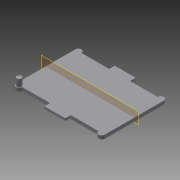
# Autodesk Inventor part: BaseTI stage insert
Saved by Autodesk Inventor 2013 (Build 170138000, 138)
## iProperties
Created: 2012-08-01
Part Number: BaseTI stage insert
Material: Generic
Document SubType Name: Modeling
Designer: kthorn
Density: 1 g/cm^3
Author: kthorn
Autodesk Inventor part; units mm, degrees
ref_plane "YZ Plane" through (0, 0, 0) normal (1, 0, 0) x (0, 1, 0)
ref_plane "XZ Plane" through (0, 0, 0) normal (0, 1, 0) x (-1, 0, 0)
ref_plane "XY Plane" through (0, 0, 0) normal (0, 0, 1) x (1, 0, 0)
sketch "Sketch1" plane through (0, 0, 0) normal (0, 0, 1) x (1, 0, 0)
  line L0 (-54.75, 42.4) -> (54.75, 42.4)
  line L1 (63.55, 42.4) -> (63.55, -42.4)
  line L2 (54.75, -42.4) -> (-54.75, -42.4)
  line L3 (-63.55, -42.4) -> (-63.55, 42.4)
  line L4 (-63.55, 42.4) -> (63.55, -42.4) construction
  line L5 (63.55, 42.4) -> (-63.55, -42.4) construction
  arc A0 (63.55, 42.4) -> (54.75, 42.4) centre (59.15, 42.4) ccw
  line L6 (-63.55, 0) -> (63.55, 0) construction
  line L7 (-8.8, 42.4) -> (-8.8, -42.4) construction
  line L8 (-63.55, 42.4) -> (-54.75, 42.4) construction
  line L9 (-54.75, 42.4) -> (-54.75, 42.4) construction
  arc A1 (-63.55, -42.4) -> (-54.75, -42.4) centre (-59.15, -42.4) ccw
  arc A2 (54.75, -42.4) -> (63.55, -42.4) centre (59.15, -42.4) ccw
  arc A3 (-54.75, 42.4) -> (-63.55, 42.4) centre (-59.15, 42.4) ccw
  point P0 (0, 0)
  dimension "d2" = 127.1
  dimension "d4" = 84.8
  dimension "d10" = 4.4
  constraints: 20 end point, 8 point on circle, 4 centre point, 4 midpoint, 4 tangent, 3 equal radius, 2 parallel, 2 point on line, 1 horizontal, 1 perpendicular
  measures "d2" distance of L3.end L1.start
  measures "d4" distance of L1.start L1.end
  measures "d10" radius of A2
extrude "Extrusion2" add sketch "Sketch1" along normal blind 5
sketch "Sketch2" plane through (0, 0, 5) normal (0, 0, 1) x (1, 0, 0)
  arc A0 (-63.55, -42.4) -> (-54.75, -42.4) centre (-59.15, -42.4) ccw projected
  circle A1 centre (-59.15, -42.4) radius 3.5
  point P0 (0, 0)
  dimension "d14" = 7
  constraints: 1 centre point, 1 coincident
  measures "d14" diameter of A1
extrude "Extrusion3" add sketch "Sketch2" along normal blind 10
sketch "Sketch3" plane through (-54.75, -42.4, 0) normal (0, -1, 0) x (1, 0, 0)
  line L0 (0, 5) -> (109.5, 5) projected
  line L1 (0, 0) -> (0, 5) projected
  line L2 (54.75, 0) -> (54.75, 1.8) construction
  line L3 (54.75, 1.8) -> (69.75, 1.8)
  line L4 (69.75, 1.8) -> (69.75, 5)
  line L5 (39.75, 5) -> (39.75, 1.8)
  line L6 (39.75, 1.8) -> (54.75, 1.8)
  dimension "d18" = 1.8
  dimension "d19" = 15
  constraints: 10 end point, 2 collinear, 2 parallel, 2 perpendicular, 2 point on line
  measures "d18" distance of L2.start L2.end
  measures "d19" distance of L5.end L2.end
extrude "Extrusion4" add sketch "Sketch3" along normal blind 8
ref_plane "Work Plane1" through (-54.75, 0, 0) normal (0, -1, 0) x (1, 0, 0)
mirror "Mirror1" about plane through (-54.75, 0, 0) normal (0, -1, 0) of "Extrusion4"
fillet "Fillet1" radius 1 4 edges at (-15, -50.4, 3.4) (15, -50.4, 3.4) (15, 50.4, 3.4) (-15, 50.4, 3.4)
body "Solid2"
